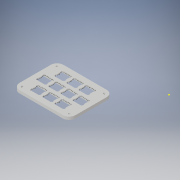
# Autodesk Inventor part: macropad-plate-01
Saved by Autodesk Inventor 2019 (Build 230136000, 136)
## iProperties
Created: 2019-01-12
Part Number: macropad-plate-01
Material: Generic
Document SubType Name: Modeling
Designer: onemo
Density: 1 g/cm^3
Appearance: Default
Author: onemo
Autodesk Inventor part; units mm, degrees
ref_plane "YZ Plane" through (0, 0, 0) normal (1, 0, 0) x (0, 1, 0)
ref_plane "XZ Plane" through (0, 0, 0) normal (0, 1, 0) x (-1, 0, 0)
ref_plane "XY Plane" through (0, 0, 0) normal (0, 0, 1) x (1, 0, 0)
sketch "Sketch1" plane through (0, 0, 0) normal (0, 1, 0) x (-1, 0, 0)
  line L0 (50.0951, 107.2477) -> (126.2953, 107.2477) construction
  line L1 (126.2953, 107.2477) -> (126.2953, 50.0978) construction
  line L2 (126.2953, 50.0978) -> (50.0951, 50.0978) construction
  line L3 (50.0951, 50.0978) -> (50.0951, 107.2477) construction
  line L4 (62.1447, 66.6247) -> (62.1447, 65.6242) construction
  line L5 (62.1447, 65.6242) -> (61.3454, 65.6242) construction
  line L6 (61.3454, 65.6242) -> (61.3454, 62.525) construction
  line L7 (61.3454, 62.525) -> (62.1447, 62.525) construction
  line L8 (62.1447, 62.525) -> (62.1447, 56.7248) construction
  line L9 (62.1447, 56.7248) -> (61.3454, 56.7248) construction
  line L10 (61.3454, 56.7248) -> (61.3454, 53.6242) construction
  line L11 (61.3454, 53.6242) -> (62.1447, 53.6242) construction
  line L12 (62.1447, 53.6242) -> (62.1447, 52.6252) construction
  line L13 (62.1447, 52.6252) -> (76.1441, 52.6252) construction
  line L14 (76.1441, 52.6252) -> (76.1441, 53.6242) construction
  line L15 (76.1441, 53.6242) -> (76.9448, 53.6242) construction
  line L16 (76.9448, 53.6242) -> (76.9448, 56.7248) construction
  line L17 (76.9448, 56.7248) -> (76.1441, 56.7248) construction
  line L18 (76.1441, 56.7248) -> (76.1441, 62.525) construction
  line L19 (76.1441, 62.525) -> (76.9448, 62.525) construction
  line L20 (76.9448, 62.525) -> (76.9448, 65.6242) construction
  line L21 (76.9448, 65.6242) -> (76.1441, 65.6242) construction
  line L22 (76.1441, 65.6242) -> (76.1441, 66.6247) construction
  line L23 (76.1441, 66.6247) -> (62.1447, 66.6247) construction
  line L24 (81.1947, 66.6247) -> (81.1947, 65.6242) construction
  line L25 (81.1947, 65.6242) -> (80.3954, 65.6242) construction
  line L26 (80.3954, 65.6242) -> (80.3954, 62.525) construction
  line L27 (80.3954, 62.525) -> (81.1947, 62.525) construction
  line L28 (81.1947, 62.525) -> (81.1947, 56.7248) construction
  line L29 (81.1947, 56.7248) -> (80.3954, 56.7248) construction
  line L30 (80.3954, 56.7248) -> (80.3954, 53.6242) construction
  line L31 (80.3954, 53.6242) -> (81.1947, 53.6242) construction
  line L32 (81.1947, 53.6242) -> (81.1947, 52.6252) construction
  line L33 (81.1947, 52.6252) -> (95.194, 52.6252) construction
  line L34 (95.194, 52.6252) -> (95.194, 53.6242) construction
  line L35 (95.194, 53.6242) -> (95.9948, 53.6242) construction
  line L36 (95.9948, 53.6242) -> (95.9948, 56.7248) construction
  line L37 (95.9948, 56.7248) -> (95.194, 56.7248) construction
  line L38 (95.194, 56.7248) -> (95.194, 62.525) construction
  line L39 (95.194, 62.525) -> (95.9948, 62.525) construction
  line L40 (95.9948, 62.525) -> (95.9948, 65.6242) construction
  line L41 (95.9948, 65.6242) -> (95.194, 65.6242) construction
  line L42 (95.194, 65.6242) -> (95.194, 66.6247) construction
  line L43 (95.194, 66.6247) -> (81.1947, 66.6247) construction
  line L44 (100.2447, 66.6247) -> (100.2447, 65.6242) construction
  line L45 (100.2447, 65.6242) -> (99.4453, 65.6242) construction
  line L46 (99.4453, 65.6242) -> (99.4453, 62.525) construction
  line L47 (99.4453, 62.525) -> (100.2447, 62.525) construction
  line L48 (100.2447, 62.525) -> (100.2447, 56.7248) construction
  line L49 (100.2447, 56.7248) -> (99.4453, 56.7248) construction
  line L50 (99.4453, 56.7248) -> (99.4453, 53.6242) construction
  line L51 (99.4453, 53.6242) -> (100.2447, 53.6242) construction
  line L52 (100.2447, 53.6242) -> (100.2447, 52.6252) construction
  line L53 (100.2447, 52.6252) -> (114.244, 52.6252) construction
  line L54 (114.244, 52.6252) -> (114.244, 53.6242) construction
  line L55 (114.244, 53.6242) -> (115.0448, 53.6242) construction
  line L56 (115.0448, 53.6242) -> (115.0448, 56.7248) construction
  line L57 (115.0448, 56.7248) -> (114.244, 56.7248) construction
  line L58 (114.244, 56.7248) -> (114.244, 62.525) construction
  line L59 (114.244, 62.525) -> (115.0448, 62.525) construction
  line L60 (115.0448, 62.525) -> (115.0448, 65.6242) construction
  line L61 (115.0448, 65.6242) -> (114.244, 65.6242) construction
  line L62 (114.244, 65.6242) -> (114.244, 66.6247) construction
  line L63 (114.244, 66.6247) -> (100.2447, 66.6247) construction
  line L64 (52.6197, 85.6747) -> (52.6197, 84.6742) construction
  line L65 (52.6197, 84.6742) -> (51.8204, 84.6742) construction
  line L66 (51.8204, 84.6742) -> (51.8204, 81.575) construction
  line L67 (51.8204, 81.575) -> (52.6197, 81.575) construction
  line L68 (52.6197, 81.575) -> (52.6197, 75.7748) construction
  line L69 (52.6197, 75.7748) -> (51.8204, 75.7748) construction
  line L70 (51.8204, 75.7748) -> (51.8204, 72.6742) construction
  line L71 (51.8204, 72.6742) -> (52.6197, 72.6742) construction
  line L72 (52.6197, 72.6742) -> (52.6197, 71.6752) construction
  line L73 (52.6197, 71.6752) -> (66.6192, 71.6752) construction
  line L74 (66.6192, 71.6752) -> (66.6192, 72.6742) construction
  line L75 (66.6192, 72.6742) -> (67.4198, 72.6742) construction
  line L76 (67.4198, 72.6742) -> (67.4198, 75.7748) construction
  line L77 (67.4198, 75.7748) -> (66.6192, 75.7748) construction
  line L78 (66.6192, 75.7748) -> (66.6192, 81.575) construction
  line L79 (66.6192, 81.575) -> (67.4198, 81.575) construction
  line L80 (67.4198, 81.575) -> (67.4198, 84.6742) construction
  line L81 (67.4198, 84.6742) -> (66.6192, 84.6742) construction
  line L82 (66.6192, 84.6742) -> (66.6192, 85.6747) construction
  line L83 (66.6192, 85.6747) -> (52.6197, 85.6747) construction
  line L84 (71.6697, 85.6747) -> (71.6697, 84.6742) construction
  line L85 (71.6697, 84.6742) -> (70.8704, 84.6742) construction
  line L86 (70.8704, 84.6742) -> (70.8704, 81.575) construction
  line L87 (70.8704, 81.575) -> (71.6697, 81.575) construction
  line L88 (71.6697, 81.575) -> (71.6697, 75.7748) construction
  line L89 (71.6697, 75.7748) -> (70.8704, 75.7748) construction
  line L90 (70.8704, 75.7748) -> (70.8704, 72.6742) construction
  line L91 (70.8704, 72.6742) -> (71.6697, 72.6742) construction
  line L92 (71.6697, 72.6742) -> (71.6697, 71.6752) construction
  line L93 (71.6697, 71.6752) -> (85.669, 71.6752) construction
  line L94 (85.669, 71.6752) -> (85.669, 72.6742) construction
  line L95 (85.669, 72.6742) -> (86.4698, 72.6742) construction
  line L96 (86.4698, 72.6742) -> (86.4698, 75.7748) construction
  line L97 (86.4698, 75.7748) -> (85.669, 75.7748) construction
  line L98 (85.669, 75.7748) -> (85.669, 81.575) construction
  line L99 (85.669, 81.575) -> (86.4698, 81.575) construction
  line L100 (86.4698, 81.575) -> (86.4698, 84.6742) construction
  line L101 (86.4698, 84.6742) -> (85.669, 84.6742) construction
  line L102 (85.669, 84.6742) -> (85.669, 85.6747) construction
  line L103 (85.669, 85.6747) -> (71.6697, 85.6747) construction
  line L104 (90.7197, 85.6747) -> (90.7197, 84.6742) construction
  line L105 (90.7197, 84.6742) -> (89.9203, 84.6742) construction
  line L106 (89.9203, 84.6742) -> (89.9203, 81.575) construction
  line L107 (89.9203, 81.575) -> (90.7197, 81.575) construction
  line L108 (90.7197, 81.575) -> (90.7197, 75.7748) construction
  line L109 (90.7197, 75.7748) -> (89.9203, 75.7748) construction
  line L110 (89.9203, 75.7748) -> (89.9203, 72.6742) construction
  line L111 (89.9203, 72.6742) -> (90.7197, 72.6742) construction
  line L112 (90.7197, 72.6742) -> (90.7197, 71.6752) construction
  line L113 (90.7197, 71.6752) -> (104.719, 71.6752) construction
  line L114 (104.719, 71.6752) -> (104.719, 72.6742) construction
  line L115 (104.719, 72.6742) -> (105.5198, 72.6742) construction
  line L116 (105.5198, 72.6742) -> (105.5198, 75.7748) construction
  line L117 (105.5198, 75.7748) -> (104.719, 75.7748) construction
  line L118 (104.719, 75.7748) -> (104.719, 81.575) construction
  line L119 (104.719, 81.575) -> (105.5198, 81.575) construction
  line L120 (105.5198, 81.575) -> (105.5198, 84.6742) construction
  line L121 (105.5198, 84.6742) -> (104.719, 84.6742) construction
  line L122 (104.719, 84.6742) -> (104.719, 85.6747) construction
  line L123 (104.719, 85.6747) -> (90.7197, 85.6747) construction
  line L124 (109.7697, 85.6747) -> (109.7697, 84.6742) construction
  line L125 (109.7697, 84.6742) -> (108.9703, 84.6742) construction
  line L126 (108.9703, 84.6742) -> (108.9703, 81.575) construction
  line L127 (108.9703, 81.575) -> (109.7697, 81.575) construction
  line L128 (109.7697, 81.575) -> (109.7697, 75.7748) construction
  line L129 (109.7697, 75.7748) -> (108.9703, 75.7748) construction
  line L130 (108.9703, 75.7748) -> (108.9703, 72.6742) construction
  line L131 (108.9703, 72.6742) -> (109.7697, 72.6742) construction
  line L132 (109.7697, 72.6742) -> (109.7697, 71.6752) construction
  line L133 (109.7697, 71.6752) -> (123.769, 71.6752) construction
  line L134 (123.769, 71.6752) -> (123.769, 72.6742) construction
  line L135 (123.769, 72.6742) -> (124.5698, 72.6742) construction
  line L136 (124.5698, 72.6742) -> (124.5698, 75.7748) construction
  line L137 (124.5698, 75.7748) -> (123.769, 75.7748) construction
  line L138 (123.769, 75.7748) -> (123.769, 81.575) construction
  line L139 (123.769, 81.575) -> (124.5698, 81.575) construction
  line L140 (124.5698, 81.575) -> (124.5698, 84.6742) construction
  line L141 (124.5698, 84.6742) -> (123.769, 84.6742) construction
  line L142 (123.769, 84.6742) -> (123.769, 85.6747) construction
  line L143 (123.769, 85.6747) -> (109.7697, 85.6747) construction
  line L144 (62.1447, 104.7247) -> (62.1447, 103.7242) construction
  line L145 (62.1447, 103.7242) -> (61.3454, 103.7242) construction
  line L146 (61.3454, 103.7242) -> (61.3454, 100.625) construction
  line L147 (61.3454, 100.625) -> (62.1447, 100.625) construction
  line L148 (62.1447, 100.625) -> (62.1447, 94.825) construction
  line L149 (62.1447, 94.825) -> (61.3454, 94.825) construction
  line L150 (61.3454, 94.825) -> (61.3454, 91.7241) construction
  line L151 (61.3454, 91.7241) -> (62.1447, 91.7241) construction
  line L152 (62.1447, 91.7241) -> (62.1447, 90.725) construction
  line L153 (62.1447, 90.725) -> (76.1441, 90.725) construction
  line L154 (76.1441, 90.725) -> (76.1441, 91.7241) construction
  line L155 (76.1441, 91.7241) -> (76.9448, 91.7241) construction
  line L156 (76.9448, 91.7241) -> (76.9448, 94.825) construction
  line L157 (76.9448, 94.825) -> (76.1441, 94.825) construction
  line L158 (76.1441, 94.825) -> (76.1441, 100.625) construction
  line L159 (76.1441, 100.625) -> (76.9448, 100.625) construction
  line L160 (76.9448, 100.625) -> (76.9448, 103.7242) construction
  line L161 (76.9448, 103.7242) -> (76.1441, 103.7242) construction
  line L162 (76.1441, 103.7242) -> (76.1441, 104.7247) construction
  line L163 (76.1441, 104.7247) -> (62.1447, 104.7247) construction
  line L164 (81.1947, 104.7247) -> (81.1947, 103.7242) construction
  line L165 (81.1947, 103.7242) -> (80.3954, 103.7242) construction
  line L166 (80.3954, 103.7242) -> (80.3954, 100.625) construction
  line L167 (80.3954, 100.625) -> (81.1947, 100.625) construction
  line L168 (81.1947, 100.625) -> (81.1947, 94.825) construction
  line L169 (81.1947, 94.825) -> (80.3954, 94.825) construction
  line L170 (80.3954, 94.825) -> (80.3954, 91.7241) construction
  line L171 (80.3954, 91.7241) -> (81.1947, 91.7241) construction
  line L172 (81.1947, 91.7241) -> (81.1947, 90.725) construction
  line L173 (81.1947, 90.725) -> (95.194, 90.725) construction
  line L174 (95.194, 90.725) -> (95.194, 91.7241) construction
  line L175 (95.194, 91.7241) -> (95.9948, 91.7241) construction
  line L176 (95.9948, 91.7241) -> (95.9948, 94.825) construction
  line L177 (95.9948, 94.825) -> (95.194, 94.825) construction
  line L178 (95.194, 94.825) -> (95.194, 100.625) construction
  line L179 (95.194, 100.625) -> (95.9948, 100.625) construction
  line L180 (95.9948, 100.625) -> (95.9948, 103.7242) construction
  line L181 (95.9948, 103.7242) -> (95.194, 103.7242) construction
  line L182 (95.194, 103.7242) -> (95.194, 104.7247) construction
  line L183 (95.194, 104.7247) -> (81.1947, 104.7247) construction
  line L184 (100.2447, 104.7247) -> (100.2447, 103.7242) construction
  line L185 (100.2447, 103.7242) -> (99.4453, 103.7242) construction
  line L186 (99.4453, 103.7242) -> (99.4453, 100.625) construction
  line L187 (99.4453, 100.625) -> (100.2447, 100.625) construction
  line L188 (100.2447, 100.625) -> (100.2447, 94.825) construction
  line L189 (100.2447, 94.825) -> (99.4453, 94.825) construction
  line L190 (99.4453, 94.825) -> (99.4453, 91.7241) construction
  line L191 (99.4453, 91.7241) -> (100.2447, 91.7241) construction
  line L192 (100.2447, 91.7241) -> (100.2447, 90.725) construction
  line L193 (100.2447, 90.725) -> (114.244, 90.725) construction
  line L194 (114.244, 90.725) -> (114.244, 91.7241) construction
  line L195 (114.244, 91.7241) -> (115.0448, 91.7241) construction
  line L196 (115.0448, 91.7241) -> (115.0448, 94.825) construction
  line L197 (115.0448, 94.825) -> (114.244, 94.825) construction
  line L198 (114.244, 94.825) -> (114.244, 100.625) construction
  line L199 (114.244, 100.625) -> (115.0448, 100.625) construction
  line L200 (115.0448, 100.625) -> (115.0448, 103.7242) construction
  line L201 (115.0448, 103.7242) -> (114.244, 103.7242) construction
  line L202 (114.244, 103.7242) -> (114.244, 104.7247) construction
  line L203 (114.244, 104.7247) -> (100.2447, 104.7247) construction
  point P0 (0, 0)
  dimension "d0" = 90
  dimension "d1" = 90
  dimension "d2" = 90
  dimension "d3" = 90
  dimension "d4" = 90
  dimension "d5" = 90
  dimension "d6" = 90
  dimension "d7" = 90
  dimension "d8" = 90
  dimension "d9" = 90
  dimension "d10" = 90
  dimension "d11" = 90
  dimension "d12" = 90
  dimension "d13" = 90
  dimension "d14" = 90
  dimension "d15" = 90
  dimension "d16" = 90
  dimension "d17" = 90
  dimension "d18" = 90
  dimension "d19" = 90
  dimension "d20" = 90
  dimension "d21" = 90
  dimension "d22" = 90
  dimension "d23" = 90
  dimension "d24" = 90
  dimension "d25" = 90
  dimension "d26" = 90
  dimension "d27" = 90
  dimension "d28" = 90
  dimension "d29" = 90
  dimension "d30" = 90
  dimension "d31" = 90
  dimension "d32" = 90
  dimension "d33" = 90
  dimension "d34" = 90
  dimension "d35" = 90
  dimension "d36" = 90
  dimension "d37" = 90
  dimension "d38" = 90
  dimension "d39" = 90
  dimension "d40" = 90
  dimension "d41" = 90
  dimension "d42" = 90
  dimension "d43" = 90
  dimension "d44" = 90
  dimension "d45" = 90
  dimension "d46" = 90
  dimension "d47" = 90
  dimension "d48" = 90
  dimension "d49" = 90
  dimension "d50" = 90
  dimension "d51" = 90
  dimension "d52" = 90
  dimension "d53" = 90
  dimension "d54" = 90
  dimension "d55" = 90
  dimension "d56" = 90
  dimension "d57" = 90
  dimension "d58" = 90
  dimension "d59" = 90
  dimension "d60" = 90
  dimension "d61" = 90
  dimension "d62" = 90
  dimension "d63" = 90
  constraints: 408 end point, 48 parallel, 1 horizontal, 1 vertical
  measures "d0" angle of L1 L125
  measures "d1" angle of L1 L127
  measures "d2" angle of L1 L129
  measures "d3" angle of L1 L131
  measures "d4" angle of L1 L121
  measures "d5" angle of L1 L119
  measures "d6" angle of L1 L117
  measures "d7" angle of L1 L115
  measures "d8" angle of L1 L185
  measures "d9" angle of L1 L187
  measures "d10" angle of L1 L189
  measures "d11" angle of L1 L191
  measures "d12" angle of L1 L45
  measures "d13" angle of L1 L47
  measures "d14" angle of L1 L49
  measures "d15" angle of L1 L51
  measures "d16" angle of L1 L123
  measures "d17" angle of L1 L113
  measures "d18" angle of L1 L181
  measures "d19" angle of L1 L179
  measures "d20" angle of L1 L177
  measures "d21" angle of L1 L175
  measures "d22" angle of L1 L41
  measures "d23" angle of L1 L39
  measures "d24" angle of L1 L37
  measures "d25" angle of L1 L35
  measures "d26" angle of L1 L105
  measures "d27" angle of L1 L107
  measures "d28" angle of L1 L109
  measures "d29" angle of L1 L111
  measures "d30" angle of L1 L183
  measures "d31" angle of L1 L173
  measures "d32" angle of L1 L43
  measures "d33" angle of L1 L33
  measures "d34" angle of L1 L101
  measures "d35" angle of L1 L99
  measures "d36" angle of L1 L97
  measures "d37" angle of L1 L95
  measures "d38" angle of L1 L165
  measures "d39" angle of L1 L167
  measures "d40" angle of L1 L169
  measures "d41" angle of L1 L171
  measures "d42" angle of L1 L25
  measures "d43" angle of L1 L27
  measures "d44" angle of L1 L29
  measures "d45" angle of L1 L31
  measures "d46" angle of L1 L103
  measures "d47" angle of L1 L93
  measures "d48" angle of L1 L161
  measures "d49" angle of L1 L159
  measures "d50" angle of L1 L157
  measures "d51" angle of L1 L155
  measures "d52" angle of L1 L21
  measures "d53" angle of L1 L19
  measures "d54" angle of L1 L17
  measures "d55" angle of L1 L15
  measures "d56" angle of L1 L85
  measures "d57" angle of L1 L87
  measures "d58" angle of L1 L89
  measures "d59" angle of L1 L91
  measures "d60" angle of L1 L163
  measures "d61" angle of L1 L153
  measures "d62" angle of L1 L23
  measures "d63" angle of L1 L13
sketch "Sketch2" plane through (0, 0, 0) normal (0, 1, 0) x (-1, 0, 0)
  line L0 (114.244, 66.6247) -> (100.2447, 66.6247) construction
  line L1 (100.2447, 66.6247) -> (100.2447, 65.6242) construction
  line L2 (100.2447, 65.6242) -> (99.4453, 65.6242) construction
  line L3 (99.4453, 65.6242) -> (99.4453, 62.525) construction
  line L4 (99.4453, 62.525) -> (100.2447, 62.525) construction
  line L5 (100.2447, 62.525) -> (100.2447, 56.7248) construction
  line L6 (100.2447, 56.7248) -> (99.4453, 56.7248) construction
  line L7 (99.4453, 56.7248) -> (99.4453, 53.6242) construction
  line L8 (99.4453, 53.6242) -> (100.2447, 53.6242) construction
  line L9 (100.2447, 53.6242) -> (100.2447, 52.6252) construction
  line L10 (100.2447, 52.6252) -> (114.244, 52.6252) construction
  line L11 (114.244, 52.6252) -> (114.244, 53.6242) construction
  line L12 (114.244, 53.6242) -> (115.0448, 53.6242) construction
  line L13 (115.0448, 53.6242) -> (115.0448, 56.7248) construction
  line L14 (115.0448, 56.7248) -> (114.244, 56.7248) construction
  line L15 (114.244, 56.7248) -> (114.244, 62.525) construction
  line L16 (114.244, 62.525) -> (115.0448, 62.525) construction
  line L17 (115.0448, 62.525) -> (115.0448, 65.6242) construction
  line L18 (115.0448, 65.6242) -> (114.244, 65.6242) construction
  line L19 (114.244, 65.6242) -> (114.244, 66.6247) construction
  line L20 (126.2953, 50.0978) -> (50.0951, 50.0978) construction
  line L21 (126.2953, 107.2477) -> (126.2953, 50.0978) construction
  line L22 (50.0951, 107.2477) -> (126.2953, 107.2477) construction
  line L23 (50.0951, 50.0978) -> (50.0951, 107.2477) construction
  line L24 (81.1947, 52.6252) -> (95.194, 52.6252) construction
  line L25 (81.1947, 53.6242) -> (81.1947, 52.6252) construction
  line L26 (80.3954, 53.6242) -> (81.1947, 53.6242) construction
  line L27 (80.3954, 56.7248) -> (80.3954, 53.6242) construction
  line L28 (81.1947, 56.7248) -> (80.3954, 56.7248) construction
  line L29 (81.1947, 62.525) -> (81.1947, 56.7248) construction
  line L30 (80.3954, 62.525) -> (81.1947, 62.525) construction
  line L31 (80.3954, 65.6242) -> (80.3954, 62.525) construction
  line L32 (81.1947, 65.6242) -> (80.3954, 65.6242) construction
  line L33 (81.1947, 66.6247) -> (81.1947, 65.6242) construction
  line L34 (95.194, 66.6247) -> (81.1947, 66.6247) construction
  line L35 (95.194, 65.6242) -> (95.194, 66.6247) construction
  line L36 (95.9948, 65.6242) -> (95.194, 65.6242) construction
  line L37 (95.9948, 62.525) -> (95.9948, 65.6242) construction
  line L38 (95.194, 62.525) -> (95.9948, 62.525) construction
  line L39 (95.194, 56.7248) -> (95.194, 62.525) construction
  line L40 (95.9948, 53.6242) -> (95.9948, 56.7248) construction
  line L41 (95.194, 53.6242) -> (95.9948, 53.6242) construction
  line L42 (95.194, 52.6252) -> (95.194, 53.6242) construction
  line L43 (76.1441, 66.6247) -> (62.1447, 66.6247) construction
  line L44 (62.1447, 66.6247) -> (62.1447, 65.6242) construction
  line L45 (62.1447, 65.6242) -> (61.3454, 65.6242) construction
  line L46 (61.3454, 65.6242) -> (61.3454, 62.525) construction
  line L47 (61.3454, 62.525) -> (62.1447, 62.525) construction
  line L48 (62.1447, 62.525) -> (62.1447, 56.7248) construction
  line L49 (62.1447, 56.7248) -> (61.3454, 56.7248) construction
  line L50 (61.3454, 56.7248) -> (61.3454, 53.6242) construction
  line L51 (61.3454, 53.6242) -> (62.1447, 53.6242) construction
  line L52 (62.1447, 53.6242) -> (62.1447, 52.6252) construction
  line L53 (62.1447, 52.6252) -> (76.1441, 52.6252) construction
  line L54 (76.1441, 52.6252) -> (76.1441, 53.6242) construction
  line L55 (76.1441, 53.6242) -> (76.9448, 53.6242) construction
  line L56 (76.9448, 53.6242) -> (76.9448, 56.7248) construction
  line L57 (76.9448, 56.7248) -> (76.1441, 56.7248) construction
  line L58 (76.1441, 56.7248) -> (76.1441, 62.525) construction
  line L59 (76.1441, 62.525) -> (76.9448, 62.525) construction
  line L60 (76.9448, 62.525) -> (76.9448, 65.6242) construction
  line L61 (76.9448, 65.6242) -> (76.1441, 65.6242) construction
  line L62 (76.1441, 65.6242) -> (76.1441, 66.6247) construction
  line L63 (123.769, 85.6747) -> (109.7697, 85.6747) construction
  line L64 (109.7697, 85.6747) -> (109.7697, 84.6742) construction
  line L65 (109.7697, 84.6742) -> (108.9703, 84.6742) construction
  line L66 (108.9703, 84.6742) -> (108.9703, 81.575) construction
  line L67 (108.9703, 81.575) -> (109.7697, 81.575) construction
  line L68 (109.7697, 81.575) -> (109.7697, 75.7748) construction
  line L69 (109.7697, 75.7748) -> (108.9703, 75.7748) construction
  line L70 (108.9703, 75.7748) -> (108.9703, 72.6742) construction
  line L71 (108.9703, 72.6742) -> (109.7697, 72.6742) construction
  line L72 (109.7697, 72.6742) -> (109.7697, 71.6752) construction
  line L73 (109.7697, 71.6752) -> (123.769, 71.6752) construction
  line L74 (123.769, 71.6752) -> (123.769, 72.6742) construction
  line L75 (123.769, 72.6742) -> (124.5698, 72.6742) construction
  line L76 (124.5698, 72.6742) -> (124.5698, 75.7748) construction
  line L77 (124.5698, 75.7748) -> (123.769, 75.7748) construction
  line L78 (123.769, 75.7748) -> (123.769, 81.575) construction
  line L79 (123.769, 81.575) -> (124.5698, 81.575) construction
  line L80 (124.5698, 81.575) -> (124.5698, 84.6742) construction
  line L81 (124.5698, 84.6742) -> (123.769, 84.6742) construction
  line L82 (123.769, 84.6742) -> (123.769, 85.6747) construction
  line L83 (104.719, 85.6747) -> (90.7197, 85.6747) construction
  line L84 (90.7197, 85.6747) -> (90.7197, 84.6742) construction
  line L85 (90.7197, 84.6742) -> (89.9203, 84.6742) construction
  line L86 (89.9203, 84.6742) -> (89.9203, 81.575) construction
  line L87 (89.9203, 81.575) -> (90.7197, 81.575) construction
  line L88 (90.7197, 81.575) -> (90.7197, 75.7748) construction
  line L89 (90.7197, 75.7748) -> (89.9203, 75.7748) construction
  line L90 (89.9203, 75.7748) -> (89.9203, 72.6742) construction
  line L91 (89.9203, 72.6742) -> (90.7197, 72.6742) construction
  line L92 (90.7197, 72.6742) -> (90.7197, 71.6752) construction
  line L93 (90.7197, 71.6752) -> (104.719, 71.6752) construction
  line L94 (104.719, 71.6752) -> (104.719, 72.6742) construction
  line L95 (104.719, 72.6742) -> (105.5198, 72.6742) construction
  line L96 (105.5198, 72.6742) -> (105.5198, 75.7748) construction
  line L97 (105.5198, 75.7748) -> (104.719, 75.7748) construction
  line L98 (104.719, 75.7748) -> (104.719, 81.575) construction
  line L99 (104.719, 81.575) -> (105.5198, 81.575) construction
  line L100 (105.5198, 81.575) -> (105.5198, 84.6742) construction
  line L101 (105.5198, 84.6742) -> (104.719, 84.6742) construction
  line L102 (104.719, 84.6742) -> (104.719, 85.6747) construction
  line L103 (85.669, 85.6747) -> (71.6697, 85.6747) construction
  line L104 (71.6697, 85.6747) -> (71.6697, 84.6742) construction
  line L105 (71.6697, 84.6742) -> (70.8704, 84.6742) construction
  line L106 (70.8704, 84.6742) -> (70.8704, 81.575) construction
  line L107 (70.8704, 81.575) -> (71.6697, 81.575) construction
  line L108 (71.6697, 81.575) -> (71.6697, 75.7748) construction
  line L109 (71.6697, 75.7748) -> (70.8704, 75.7748) construction
  line L110 (70.8704, 75.7748) -> (70.8704, 72.6742) construction
  line L111 (70.8704, 72.6742) -> (71.6697, 72.6742) construction
  line L112 (71.6697, 72.6742) -> (71.6697, 71.6752) construction
  line L113 (71.6697, 71.6752) -> (85.669, 71.6752) construction
  line L114 (85.669, 71.6752) -> (85.669, 72.6742) construction
  line L115 (85.669, 72.6742) -> (86.4698, 72.6742) construction
  line L116 (86.4698, 72.6742) -> (86.4698, 75.7748) construction
  line L117 (86.4698, 75.7748) -> (85.669, 75.7748) construction
  line L118 (85.669, 75.7748) -> (85.669, 81.575) construction
  line L119 (85.669, 81.575) -> (86.4698, 81.575) construction
  line L120 (86.4698, 81.575) -> (86.4698, 84.6742) construction
  line L121 (86.4698, 84.6742) -> (85.669, 84.6742) construction
  line L122 (85.669, 84.6742) -> (85.669, 85.6747) construction
  line L123 (66.6192, 85.6747) -> (52.6197, 85.6747) construction
  line L124 (52.6197, 85.6747) -> (52.6197, 84.6742) construction
  line L125 (52.6197, 84.6742) -> (51.8204, 84.6742) construction
  line L126 (51.8204, 84.6742) -> (51.8204, 81.575) construction
  line L127 (51.8204, 81.575) -> (52.6197, 81.575) construction
  line L128 (52.6197, 81.575) -> (52.6197, 75.7748) construction
  line L129 (52.6197, 75.7748) -> (51.8204, 75.7748) construction
  line L130 (51.8204, 75.7748) -> (51.8204, 72.6742) construction
  line L131 (51.8204, 72.6742) -> (52.6197, 72.6742) construction
  line L132 (52.6197, 72.6742) -> (52.6197, 71.6752) construction
  line L133 (52.6197, 71.6752) -> (66.6192, 71.6752) construction
  line L134 (66.6192, 71.6752) -> (66.6192, 72.6742) construction
  line L135 (66.6192, 72.6742) -> (67.4198, 72.6742) construction
  line L136 (67.4198, 72.6742) -> (67.4198, 75.7748) construction
  line L137 (67.4198, 75.7748) -> (66.6192, 75.7748) construction
  line L138 (66.6192, 75.7748) -> (66.6192, 81.575) construction
  line L139 (66.6192, 81.575) -> (67.4198, 81.575) construction
  line L140 (67.4198, 81.575) -> (67.4198, 84.6742) construction
  line L141 (67.4198, 84.6742) -> (66.6192, 84.6742) construction
  line L142 (66.6192, 84.6742) -> (66.6192, 85.6747) construction
  line L143 (114.244, 104.7247) -> (100.2447, 104.7247) construction
  line L144 (100.2447, 104.7247) -> (100.2447, 103.7242) construction
  line L145 (100.2447, 103.7242) -> (99.4453, 103.7242) construction
  line L146 (99.4453, 103.7242) -> (99.4453, 100.625) construction
  line L147 (99.4453, 100.625) -> (100.2447, 100.625) construction
  line L148 (100.2447, 100.625) -> (100.2447, 94.825) construction
  line L149 (100.2447, 94.825) -> (99.4453, 94.825) construction
  line L150 (99.4453, 94.825) -> (99.4453, 91.7241) construction
  line L151 (99.4453, 91.7241) -> (100.2447, 91.7241) construction
  line L152 (100.2447, 91.7241) -> (100.2447, 90.725) construction
  line L153 (100.2447, 90.725) -> (114.244, 90.725) construction
  line L154 (114.244, 90.725) -> (114.244, 91.7241) construction
  line L155 (114.244, 91.7241) -> (115.0448, 91.7241) construction
  line L156 (115.0448, 91.7241) -> (115.0448, 94.825) construction
  line L157 (115.0448, 94.825) -> (114.244, 94.825) construction
  line L158 (114.244, 94.825) -> (114.244, 100.625) construction
  line L159 (114.244, 100.625) -> (115.0448, 100.625) construction
  line L160 (115.0448, 100.625) -> (115.0448, 103.7242) construction
  line L161 (115.0448, 103.7242) -> (114.244, 103.7242) construction
  line L162 (114.244, 103.7242) -> (114.244, 104.7247) construction
  line L163 (80.3954, 103.7242) -> (80.3954, 100.625) construction
  line L164 (80.3954, 100.625) -> (81.1947, 100.625) construction
  line L165 (81.1947, 100.625) -> (81.1947, 94.825) construction
  line L166 (81.1947, 94.825) -> (80.3954, 94.825) construction
  line L167 (80.3954, 94.825) -> (80.3954, 91.7241) construction
  line L168 (80.3954, 91.7241) -> (81.1947, 91.7241) construction
  line L169 (81.1947, 91.7241) -> (81.1947, 90.725) construction
  line L170 (81.1947, 90.725) -> (95.194, 90.725) construction
  line L171 (95.194, 90.725) -> (95.194, 91.7241) construction
  line L172 (95.194, 91.7241) -> (95.9948, 91.7241) construction
  line L173 (95.9948, 91.7241) -> (95.9948, 94.825) construction
  line L174 (95.9948, 94.825) -> (95.194, 94.825) construction
  line L175 (95.194, 94.825) -> (95.194, 100.625) construction
  line L176 (95.194, 100.625) -> (95.9948, 100.625) construction
  line L177 (95.9948, 100.625) -> (95.9948, 103.7242) construction
  line L178 (95.9948, 103.7242) -> (95.194, 103.7242) construction
  line L179 (95.194, 103.7242) -> (95.194, 104.7247) construction
  line L180 (95.194, 104.7247) -> (81.1947, 104.7247) construction
  line L181 (76.1441, 104.7247) -> (62.1447, 104.7247) construction
  line L182 (62.1447, 104.7247) -> (62.1447, 103.7242) construction
  line L183 (62.1447, 103.7242) -> (61.3454, 103.7242) construction
  line L184 (61.3454, 103.7242) -> (61.3454, 100.625) construction
  line L185 (61.3454, 100.625) -> (62.1447, 100.625) construction
  line L186 (62.1447, 100.625) -> (62.1447, 94.825) construction
  line L187 (62.1447, 94.825) -> (61.3454, 94.825) construction
  line L188 (61.3454, 94.825) -> (61.3454, 91.7241) construction
  line L189 (61.3454, 91.7241) -> (62.1447, 91.7241) construction
  line L190 (62.1447, 91.7241) -> (62.1447, 90.725) construction
  line L191 (62.1447, 90.725) -> (76.1441, 90.725) construction
  line L192 (76.1441, 90.725) -> (76.1441, 91.7241) construction
  line L193 (76.1441, 91.7241) -> (76.9448, 91.7241) construction
  line L194 (76.9448, 91.7241) -> (76.9448, 94.825) construction
  line L195 (76.9448, 94.825) -> (76.1441, 94.825) construction
  line L196 (76.1441, 94.825) -> (76.1441, 100.625) construction
  line L197 (76.1441, 100.625) -> (76.9448, 100.625) construction
  line L198 (76.9448, 100.625) -> (76.9448, 103.7242) construction
  line L199 (76.9448, 103.7242) -> (76.1441, 103.7242) construction
  line L200 (76.1441, 103.7242) -> (76.1441, 104.7247) construction
  line L201 (115.0448, 53.6242) -> (99.4453, 53.6242)
  line L202 (99.4453, 53.6242) -> (99.4453, 56.7248)
  line L203 (99.4453, 56.7248) -> (115.0448, 56.7248)
  line L204 (115.0448, 56.7248) -> (115.0448, 53.6242)
  line L205 (115.0448, 62.525) -> (99.4453, 62.525)
  line L206 (99.4453, 62.525) -> (99.4453, 65.6242)
  line L207 (99.4453, 65.6242) -> (115.0448, 65.6242)
  line L208 (115.0448, 65.6242) -> (115.0448, 62.525)
  line L209 (114.244, 52.6252) -> (100.2447, 52.6252)
  line L210 (100.2447, 52.6252) -> (100.2447, 66.6247)
  line L211 (100.2447, 66.6247) -> (114.244, 66.6247)
  line L212 (114.244, 66.6247) -> (114.244, 52.6252)
  line L213 (95.9948, 62.525) -> (80.3954, 62.525)
  line L214 (80.3954, 62.525) -> (80.3954, 65.6242)
  line L215 (80.3954, 65.6242) -> (95.9948, 65.6242)
  line L216 (95.9948, 65.6242) -> (95.9948, 62.525)
  line L217 (95.9948, 53.6242) -> (80.3954, 53.6242)
  line L218 (80.3954, 53.6242) -> (80.3954, 56.7248)
  line L219 (80.3954, 56.7248) -> (95.9948, 56.7248)
  line L220 (95.9948, 56.7248) -> (95.9948, 53.6242)
  line L221 (95.194, 52.6252) -> (81.1947, 52.6252)
  line L222 (81.1947, 52.6252) -> (81.1947, 66.6247)
  line L223 (81.1947, 66.6247) -> (95.194, 66.6247)
  line L224 (95.194, 66.6247) -> (95.194, 52.6252)
  line L225 (76.1441, 52.6252) -> (62.1447, 52.6252)
  line L226 (62.1447, 52.6252) -> (62.1447, 66.6247)
  line L227 (62.1447, 66.6247) -> (76.1441, 66.6247)
  line L228 (76.1441, 66.6247) -> (76.1441, 52.6252)
  line L229 (76.9448, 53.6242) -> (61.3454, 53.6242)
  line L230 (61.3454, 53.6242) -> (61.3454, 56.7248)
  line L231 (61.3454, 56.7248) -> (76.9448, 56.7248)
  line L232 (76.9448, 56.7248) -> (76.9448, 53.6242)
  line L233 (61.3454, 62.525) -> (76.9448, 62.525)
  line L234 (76.9448, 62.525) -> (76.9448, 65.6242)
  line L235 (76.9448, 65.6242) -> (61.3454, 65.6242)
  line L236 (61.3454, 65.6242) -> (61.3454, 62.525)
  line L237 (109.7697, 85.6747) -> (123.769, 85.6747)
  line L238 (123.769, 85.6747) -> (123.769, 71.6752)
  line L239 (123.769, 71.6752) -> (109.7697, 71.6752)
  line L240 (109.7697, 71.6752) -> (109.7697, 85.6747)
  line L241 (124.5698, 72.6742) -> (108.9703, 72.6742)
  line L242 (108.9703, 72.6742) -> (108.9703, 75.7748)
  line L243 (108.9703, 75.7748) -> (124.5698, 75.7748)
  line L244 (124.5698, 75.7748) -> (124.5698, 72.6742)
  line L245 (108.9703, 81.575) -> (124.5698, 81.575)
  line L246 (124.5698, 81.575) -> (124.5698, 84.6742)
  line L247 (124.5698, 84.6742) -> (108.9703, 84.6742)
  line L248 (108.9703, 84.6742) -> (108.9703, 81.575)
  line L249 (105.5198, 72.6742) -> (89.9203, 72.6742)
  line L250 (89.9203, 72.6742) -> (89.9203, 75.7748)
  line L251 (89.9203, 75.7748) -> (105.5198, 75.7748)
  line L252 (105.5198, 75.7748) -> (105.5198, 72.6742)
  line L253 (105.5198, 81.575) -> (89.9203, 81.575)
  line L254 (89.9203, 81.575) -> (89.9203, 84.6742)
  line L255 (89.9203, 84.6742) -> (105.5198, 84.6742)
  line L256 (105.5198, 84.6742) -> (105.5198, 81.575)
  line L257 (104.719, 71.6752) -> (90.7197, 71.6752)
  line L258 (90.7197, 71.6752) -> (90.7197, 85.6747)
  line L259 (90.7197, 85.6747) -> (104.719, 85.6747)
  line L260 (104.719, 85.6747) -> (104.719, 71.6752)
  line L261 (85.669, 71.6752) -> (71.6697, 71.6752)
  line L262 (71.6697, 71.6752) -> (71.6697, 85.6747)
  line L263 (71.6697, 85.6747) -> (85.669, 85.6747)
  line L264 (85.669, 85.6747) -> (85.669, 71.6752)
  line L265 (70.8704, 72.6742) -> (86.4698, 72.6742)
  line L266 (86.4698, 72.6742) -> (86.4698, 75.7748)
  line L267 (86.4698, 75.7748) -> (70.8704, 75.7748)
  line L268 (70.8704, 75.7748) -> (70.8704, 72.6742)
  line L269 (86.4698, 81.575) -> (70.8704, 81.575)
  line L270 (70.8704, 81.575) -> (70.8704, 84.6742)
  line L271 (70.8704, 84.6742) -> (86.4698, 84.6742)
  line L272 (86.4698, 84.6742) -> (86.4698, 81.575)
  line L273 (67.4198, 72.6742) -> (51.8204, 72.6742)
  line L274 (51.8204, 72.6742) -> (51.8204, 75.7748)
  line L275 (51.8204, 75.7748) -> (67.4198, 75.7748)
  line L276 (67.4198, 75.7748) -> (67.4198, 72.6742)
  line L277 (51.8204, 81.575) -> (67.4198, 81.575)
  line L278 (67.4198, 81.575) -> (67.4198, 84.6742)
  line L279 (67.4198, 84.6742) -> (51.8204, 84.6742)
  line L280 (51.8204, 84.6742) -> (51.8204, 81.575)
  line L281 (66.6192, 71.6752) -> (52.6197, 71.6752)
  line L282 (52.6197, 71.6752) -> (52.6197, 85.6747)
  line L283 (52.6197, 85.6747) -> (66.6192, 85.6747)
  line L284 (66.6192, 85.6747) -> (66.6192, 71.6752)
  line L285 (114.244, 90.725) -> (100.2447, 90.725)
  line L286 (100.2447, 90.725) -> (100.2447, 104.7247)
  line L287 (100.2447, 104.7247) -> (114.244, 104.7247)
  line L288 (114.244, 104.7247) -> (114.244, 90.725)
  line L289 (99.4453, 91.7241) -> (115.0448, 91.7241)
  line L290 (115.0448, 91.7241) -> (115.0448, 94.825)
  line L291 (115.0448, 94.825) -> (99.4453, 94.825)
  line L292 (99.4453, 94.825) -> (99.4453, 91.7241)
  line L293 (115.0448, 100.625) -> (99.4453, 100.625)
  line L294 (99.4453, 100.625) -> (99.4453, 103.7242)
  line L295 (99.4453, 103.7242) -> (115.0448, 103.7242)
  line L296 (115.0448, 103.7242) -> (115.0448, 100.625)
  line L297 (95.9948, 91.7241) -> (80.3954, 91.7241)
  line L298 (80.3954, 91.7241) -> (80.3954, 94.825)
  line L299 (80.3954, 94.825) -> (95.9948, 94.825)
  line L300 (95.9948, 94.825) -> (95.9948, 91.7241)
  line L301 (95.9948, 100.625) -> (80.3954, 100.625)
  line L302 (80.3954, 100.625) -> (80.3954, 103.7242)
  line L303 (80.3954, 103.7242) -> (95.9948, 103.7242)
  line L304 (95.9948, 103.7242) -> (95.9948, 100.625)
  line L305 (95.194, 90.725) -> (81.1947, 90.725)
  line L306 (81.1947, 90.725) -> (81.1947, 104.7247)
  line L307 (81.1947, 104.7247) -> (95.194, 104.7247)
  line L308 (95.194, 104.7247) -> (95.194, 90.725)
  line L309 (76.9448, 91.7241) -> (61.3454, 91.7241)
  line L310 (61.3454, 91.7241) -> (61.3454, 94.825)
  line L311 (61.3454, 94.825) -> (76.9448, 94.825)
  line L312 (76.9448, 94.825) -> (76.9448, 91.7241)
  line L313 (61.3454, 100.625) -> (76.9448, 100.625)
  line L314 (76.9448, 100.625) -> (76.9448, 103.7242)
  line L315 (76.9448, 103.7242) -> (61.3454, 103.7242)
  line L316 (61.3454, 103.7242) -> (61.3454, 100.625)
  line L317 (76.1441, 104.7247) -> (62.1447, 104.7247)
  line L318 (62.1447, 104.7247) -> (62.1447, 90.725)
  line L319 (62.1447, 90.725) -> (76.1441, 90.725)
  line L320 (76.1441, 90.725) -> (76.1441, 104.7247)
  line L321 (132.2953, 44.0978) -> (44.0951, 44.0978)
  line L322 (44.0951, 44.0978) -> (44.0951, 113.2477)
  line L323 (44.0951, 113.2477) -> (132.2953, 113.2477)
  line L324 (132.2953, 113.2477) -> (132.2953, 44.0978)
  point P0 (0, 0)
  dimension "d766" = 6
  dimension "d767" = 6
  dimension "d768" = 6
  dimension "d769" = 6
  constraints: 248 end point, 62 parallel, 31 horizontal, 31 perpendicular
  measures "d766" distance between parallel lines of L324 L21
  measures "d767" distance between parallel lines of L23 L322
  measures "d768" distance between parallel lines of L22 L323
  measures "d769" distance between parallel lines of L321 L20
extrude "Extrusion1" add sketch "Sketch2" along normal blind 1.5
fillet "Fillet2" radius 10 4 edges at (-132.2953, 0.75, 44.0978) (-44.0951, 0.75, 44.0978) (-44.0951, 0.75, 113.2477) (-132.2953, 0.75, 113.2477)
sketch "Sketch5" plane through (0, 0, 0) normal (0, -1, 0) x (1, 0, 0)
  circle A0 centre (-51.0951, 51.0978) radius 1.5
  circle A1 centre (-125.2953, 51.0978) radius 1.5
  circle A2 centre (-51.0951, 106.2477) radius 1.5
  circle A3 centre (-125.2953, 106.2477) radius 1.5
  line L0 (-132.2953, 103.2477) -> (-132.2953, 54.0978) projected
  line L1 (-54.0951, 113.2477) -> (-122.2953, 113.2477) projected
  line L2 (-44.0951, 54.0978) -> (-44.0951, 103.2477) projected
  line L3 (-122.2953, 44.0978) -> (-54.0951, 44.0978) projected
  point P0 (0, 0)
  dimension "d790" = 7
  dimension "d791" = 7
  dimension "d792" = 7
  dimension "d793" = 7
  dimension "d794" = 7
  dimension "d795" = 7
  dimension "d796" = 7
  dimension "d797" = 7
  dimension "d798" = 3
  dimension "d799" = 3
  dimension "d800" = 3
  dimension "d801" = 3
  constraints: 4 centre point
  measures "d790" distance from line of L0 A3.centre
  measures "d791" distance from line of A3.centre L1
  measures "d792" distance from line of L1 A2.centre
  measures "d793" distance from line of A2.centre L2
  measures "d794" distance from line of L2 A0.centre
  measures "d795" distance from line of L3 A0.centre
  measures "d796" distance from line of L0 A1.centre
  measures "d797" distance from line of L3 A1.centre
  measures "d798" diameter of A0
  measures "d799" diameter of A1
  measures "d800" diameter of A2
  measures "d801" diameter of A3
hole "Hole1" at (-51.0951, 0, 51.0978) at (-125.2953, 0, 51.0978) at (-125.2953, 0, 106.2477) at (-51.0951, 0, 106.2477) direction (0, 1, 0) diameter 3 end through all
sketch "Sketch6" plane through (0, 0, 0) normal (0, -1, 0) x (1, 0, 0)
  line L0 (-54.0951, 113.2477) -> (-122.2953, 113.2477) projected
  line L1 (-122.2953, 44.0978) -> (-54.0951, 44.0978) projected
  line L2 (-44.0951, 54.0978) -> (-44.0951, 103.2477) projected
  arc A0 (-54.0951, 44.0978) -> (-44.0951, 54.0978) centre (-54.0951, 54.0978) ccw projected
  arc A1 (-44.0951, 103.2477) -> (-54.0951, 113.2477) centre (-54.0951, 103.2477) ccw projected
  arc A2 (-122.2953, 113.2477) -> (-132.2953, 103.2477) centre (-122.2953, 103.2477) ccw projected
  line L3 (-132.2953, 103.2477) -> (-132.2953, 54.0978) projected
  arc A3 (-132.2953, 54.0978) -> (-122.2953, 44.0978) centre (-122.2953, 54.0978) ccw projected
  line L4 (-44.0951, 103.2477) -> (-44.0951, 54.0978) projected
  line L5 (-44.0951, 89.7477) -> (-132.2953, 89.7477)
  line L6 (-132.2953, 89.7477) -> (-132.2953, 86.7477)
  line L7 (-132.2953, 86.7477) -> (-44.0951, 86.7477)
  line L8 (-44.0951, 86.7477) -> (-44.0951, 89.7477)
  line L9 (-132.2953, 70.7477) -> (-44.0951, 70.7477)
  line L10 (-44.0951, 70.7477) -> (-44.0951, 67.7477)
  line L11 (-44.0951, 67.7477) -> (-132.2953, 67.7477)
  line L12 (-132.2953, 67.7477) -> (-132.2953, 70.7477)
  line L13 (-118.2953, 89.7477) -> (-118.2953, 106.2477)
  line L14 (-118.2953, 106.2477) -> (-58.0951, 106.2477)
  line L15 (-58.0951, 106.2477) -> (-58.0951, 89.7477)
  line L16 (-118.2953, 67.7477) -> (-118.2953, 51.0978)
  line L17 (-118.2953, 51.0978) -> (-58.0951, 51.0978)
  line L18 (-58.0951, 51.0978) -> (-58.0951, 67.7477)
  line L19 (-48.0951, 86.7477) -> (-48.0951, 85.0854)
  line L20 (-48.0951, 85.0854) -> (-48.0951, 70.7477)
  line L21 (-128.2953, 86.7477) -> (-128.2953, 70.7477)
  circle A4 centre (-51.0951, 51.0978) radius 1.5 projected
  circle A5 centre (-125.2953, 51.0978) radius 1.5 projected
  circle A6 centre (-125.2953, 106.2477) radius 1.5 projected
  circle A7 centre (-51.0951, 106.2477) radius 1.5 projected
  line L22 (-44.0951, 86.7477) -> (-44.0951, 70.7477)
  line L23 (-48.0951, 70.7477) -> (-48.0951, 86.7477)
  line L24 (-44.0951, 67.7477) -> (-58.0951, 67.7477)
  line L25 (-44.0951, 67.7477) -> (-44.0951, 54.0978)
  line L26 (-54.0951, 44.0978) -> (-122.2953, 44.0978)
  line L27 (-132.2953, 54.0978) -> (-132.2953, 67.7477)
  line L28 (-132.2953, 67.7477) -> (-44.0951, 67.7477)
  line L29 (-58.0951, 67.7477) -> (-58.0951, 51.0978)
  line L30 (-58.0951, 51.0978) -> (-118.2953, 51.0978)
  line L31 (-118.2953, 51.0978) -> (-118.2953, 67.7477)
  arc A8 (-54.0951, 44.0978) -> (-44.0951, 54.0978) centre (-54.0951, 54.0978) ccw
  arc A9 (-132.2953, 54.0978) -> (-122.2953, 44.0978) centre (-122.2953, 54.0978) ccw
  line L32 (-58.0951, 67.7477) -> (-118.2953, 67.7477)
  line L33 (-118.2953, 67.7477) -> (-118.2953, 51.0978)
  line L34 (-118.2953, 51.0978) -> (-58.0951, 51.0978)
  line L35 (-58.0951, 51.0978) -> (-58.0951, 67.7477)
  line L36 (-58.0951, 67.7477) -> (-44.0951, 67.7477)
  line L37 (-44.0951, 67.7477) -> (-44.0951, 54.0978)
  arc A10 (-54.0951, 44.0978) -> (-44.0951, 54.0978) centre (-54.0951, 54.0978) ccw
  circle A11 centre (-51.0951, 51.0978) radius 1.5
  circle A12 centre (-125.2953, 51.0978) radius 1.5
  point P0 (0, 0)
  dimension "d809" = 16
  dimension "d810" = 3
  dimension "d811" = 3
  dimension "d812" = 23.5
  dimension "d813" = 23.6499
  dimension "d814" = 14
  dimension "d815" = 14
  dimension "d816" = 7
  dimension "d817" = 7
  dimension "d818" = 14
  dimension "d819" = 14
  dimension "d820" = 4
  dimension "d821" = 4
  constraints: 66 end point, 17 point on line, 10 collinear, 9 perpendicular, 6 parallel, 6 point on circle, 5 centre point, 3 concentric, 3 horizontal, 2 coincident, 2 tangent, 1 vertical
  measures "d809" distance between parallel lines of L9 L7
  measures "d810" distance between parallel lines of L11 L9
  measures "d811" distance between parallel lines of L5 L7
  measures "d812" distance between parallel lines of L0 L5
  measures "d813" distance between parallel lines of L1 L11
  measures "d814" distance between parallel lines of L3 L13
  measures "d815" distance between parallel lines of L3 L16
  measures "d816" distance between parallel lines of L0 L14
  measures "d817" distance between parallel lines of L17 L1
  measures "d818" distance between parallel lines of L2 L15
  measures "d819" distance between parallel lines of L2 L18
  measures "d820" distance between parallel lines of L3 L21
  measures "d821" distance between parallel lines of L2 L20
extrude "Extrusion4" add sketch "Sketch6" along normal blind 3 contours A1 L2 L5 L15 L14 L13 L3 A2 L0 | L2 L7 L3 L5 | L2 L9 L20 L19 L7 | L7 L21 L9 L3 | L2 L11 L3 L9 | L2 A0 L1 A3 L3 L11 L16 L17 L18
equation "\"d766\" = d767"
equation "\"d768\" = d767"
equation "\"d769\" = d767"
equation "\"d790\" = d794"
equation "\"d791\" = d795"
equation "\"d792\" = d795"
equation "\"d793\" = d794"
equation "\"d796\" = d794"
equation "\"d797\" = d795"
equation "\"d799\" = d798"
equation "\"d800\" = d798"
equation "\"d801\" = d798"
equation "\"d810\" = d811"
equation "\"d818\" = d814"
body "Solid1"
